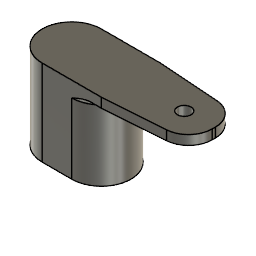
Shaft_Sensor_Holder_Noris (Autodesk Fusion 360 design; units mm, degrees)
Autodesk Fusion 360 part; units mm, degrees
sketch "Skizze1" plane through (0, 0, 0) normal (0, 0, 1) x (1, 0, 0)
  line L0 (0, 0) -> (15, 0)
  line L1 (15, 0) -> (15, 10)
  line L2 (15, 10) -> (0, 10)
  line L3 (0, 10) -> (0, 0)
  dimension "d1" = 15
  dimension "d2" = 10
  constraint horizontal L0
  constraint vertical L1
  constraint horizontal L2
  constraint vertical L3
  constraint coincident L0.start L3.end
  measures "d1" distance of L0.start L0.end
  measures "d2" distance of L0.start L2.end
extrude "Extrusion1" add sketch "Skizze1" along normal blind 12.9
sketch "Skizze2" plane through (0, 0, 12.9) normal (0, 0, 1) x (-1, 0, 0)
  line L0 (0, -10) -> (0, 0)
  line L1 (0, 0) -> (-15, 0)
  line L2 (-15, 0) -> (-15, -10)
  line L3 (-15, -10) -> (0, -10)
  circle A0 centre (-24, -5) radius 1.15
  line L4 (0, -10) -> (-15, -10)
  line L5 (-15, -10) -> (-29, -9)
  line L6 (-29, -9) -> (-29, -1)
  line L7 (-29, -1) -> (-15, 0)
  dimension "Bohrung" = 2.3
  dimension "d8" = 8
  dimension "d9" = 1
  dimension "d12" = 5
  dimension "d21" = 4
  dimension "d22" = 10
  constraint coincident L0.start L3.end
  constraint coincident L2.end L3.start
  constraint parallel L2 L6
  constraint coincident L1.end L2.start
  measures "Bohrung" diameter of A0
  measures "d8" distance of L5.end L6.end
  measures "d9" distance of L4 L5.end
  measures "d12" distance of A0.centre L6
  measures "d21" vertical distance of A0.centre L5.end
  measures "d22" distance of L0.start L0.end
extrude "Extrusion2" add sketch "Skizze2" along normal blind 1.6
fillet "Abrundung1" radius 4 2 edges at (29, 9, 13.7) (29, 1, 13.7)
fillet "Abrundung2" radius 5 4 edges at (15, 10, 6.45) (15, 0, 6.45) (0, 0, 7.25) (0, 10, 7.25)
fillet "Abrundung3" radius 1 1 edges at (15, 5, 12.9)
equation "Abstand_Sensor = 12.9 mm" comment "Hier lässt sich die Länge des Abstandshalters einstellen. (Gemessen von Unterkante Abstandshalter bis Rückseite Sensor)  Here you can adjust the length of the spacer. (Measured form bottom ede of the spacher to the backside of the sensor PCB)"
equation "Bohrung = 2.3 mm" comment "Hier lässt sich der Durchmesser für das Schraubloch einstellen.  Here you can adjust the diameter of the hole for the M2 screw."
equation "Länge_Arm = 29 mm" comment "Hier lässt sich die Länge des Arms einstellen an dem der Sensor angeschraubt wird. Here you can adjust the length of the arm on which the sensor is screwed."
equation "Armdicke = 1.6 mm" comment "Ich habe den Arm genau so dick gemacht wie das PCB des Sensors."
